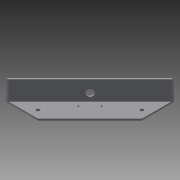
# Autodesk Inventor part: body_inner_L_clamp
Saved by Autodesk Inventor 2015 (Build 190159000, 159)
## iProperties
Created: 2017-09-26
Part Number: body_inner_L_clamp
Material: Generic
Document SubType Name: Modeling
Designer: Anshul
Density: 1 g/cm^3
Appearance: Default
Author: Anshul
Autodesk Inventor part; units mm, degrees
ref_plane "YZ Plane" through (0, 0, 0) normal (1, 0, 0) x (0, 1, 0)
ref_plane "XZ Plane" through (0, 0, 0) normal (0, 1, 0) x (-1, 0, 0)
ref_plane "XY Plane" through (0, 0, 0) normal (0, 0, 1) x (1, 0, 0)
sketch "Sketch1" plane through (0, 0, 0) normal (0, 1, 0) x (-1, 0, 0)
  line L0 (0, 0) -> (0, -650)
  line L1 (0, -650) -> (650, -650)
  line L2 (650, -650) -> (650, 0)
  line L3 (650, 0) -> (0, 0)
  line L4 (0, 0) -> (3, 0)
  line L5 (3, 0) -> (3, -650)
  line L6 (3, -650) -> (0, -650)
  line L7 (0, -650) -> (0, -647)
  line L8 (0, -647) -> (650, -647)
  line L9 (650, -647) -> (650, -650)
  line L10 (650, -650) -> (647, -650)
  line L11 (647, -650) -> (647, 0)
  line L12 (647, 0) -> (650, 0)
  line L13 (650, 0) -> (650, -3)
  line L14 (650, -3) -> (0, -3)
  line L15 (0, -3) -> (0, 0)
  line L16 (0, 0) -> (0, -37)
  line L17 (0, -37) -> (650, -37)
  line L18 (650, -37) -> (650, 0)
  line L19 (650, 0) -> (613, 0)
  line L20 (613, 0) -> (613, -650)
  line L21 (613, -650) -> (650, -650)
  line L22 (650, -650) -> (650, -613)
  line L23 (650, -613) -> (0, -613)
  line L24 (0, -613) -> (0, -650)
  line L25 (0, -650) -> (37, -650)
  line L26 (37, -650) -> (37, 0)
  line L27 (37, 0) -> (0, 0)
  line L28 (0, 0) -> (650, -650)
  line L29 (650, 0) -> (0, -650)
  line L30 (37, -3) -> (3, -37)
  line L31 (20, -20) -> (75.1543, -75.1543)
  line L32 (75.1543, -75.1543) -> (3, -147.3087)
  line L33 (75.1543, -75.1543) -> (147.3087, -3)
  line L34 (75.1543, -75.1543) -> (48.9914, -48.9914)
  line L35 (48.9914, -48.9914) -> (3, -94.9828)
  line L36 (48.9914, -48.9914) -> (94.9828, -3)
  line L37 (75.1543, -75.1543) -> (77.2756, -77.2756)
  line L38 (77.2756, -77.2756) -> (3, -151.5513)
  line L39 (77.2756, -77.2756) -> (151.5513, -3)
  line L40 (75.1543, -75.1543) -> (68.0833, -68.0833)
  line L41 (68.0833, -68.0833) -> (57.8302, -78.3363)
  line L42 (68.0833, -68.0833) -> (78.3363, -57.8302)
  circle A0 centre (78.3363, -57.8302) radius 1.5
  circle A1 centre (57.8302, -78.3363) radius 1.5
  line L43 (3, -147.3087) -> (3, -94.9828)
  line L44 (147.3087, -3) -> (94.9828, -3)
  line L45 (121.1457, -3) -> (3, -121.1457)
  circle A2 centre (62.0729, -62.0729) radius 65
  circle A3 centre (108.0348, -16.1109) radius 3
  circle A4 centre (16.1109, -108.0348) radius 3
  dimension "d0" = 650
  dimension "d1" = 650
  dimension "d2" = 650
  dimension "d3" = 3
  dimension "d4" = 650
  dimension "d5" = 3
  dimension "d6" = 3
  dimension "d7" = 650
  dimension "d8" = 3
  dimension "d9" = 650
  dimension "d10" = 37
  dimension "d11" = 650
  dimension "d12" = 37
  dimension "d13" = 650
  dimension "d14" = 37
  dimension "d15" = 650
  dimension "d16" = 37
  dimension "d17" = 650
  dimension "d18" = 78
  dimension "d19" = 37
  dimension "d20" = 3
  dimension "d21" = 10
  dimension "d22" = 14.5
  dimension "d23" = 14.5
  dimension "d24" = 3
  dimension "d25" = 3
  dimension "d26" = 130
  dimension "d27" = 6
  dimension "d28" = 6
  constraints: 92 end point, 35 point on line, 8 perpendicular, 5 centre point, 5 collinear, 4 midpoint, 2 coincident, 2 point on circle, 1 parallel, 1 vertical
  measures "d0" distance of L0.start L0.end
  measures "d1" distance of L0.end L1.end
  measures "d2" distance of L1.end L2.end
  measures "d3" distance of L0.start L4.end
  measures "d4" distance of L4.end L5.end
  measures "d5" distance of L0.end L7.end
  measures "d6" distance of L1.end L10.end
  measures "d7" distance of L10.end L11.end
  measures "d8" distance of L2.end L13.end
  measures "d9" distance of L13.end L14.end
  measures "d10" distance of L0.start L16.end
  measures "d11" distance of L16.end L17.end
  measures "d12" distance of L2.end L19.end
  measures "d13" distance of L19.end L20.end
  measures "d14" distance of L1.end L22.end
  measures "d15" distance of L22.end L23.end
  measures "d16" distance of L0.end L25.end
  measures "d17" distance of L25.end L26.end
  measures "d18" distance of L31.start L31.end
  measures "d19" distance of L31.end L34.end
  measures "d20" distance of L31.end L37.end
  measures "d21" distance of L31.end L40.end
  measures "d22" distance of L40.end L41.end
  measures "d23" distance of L40.end L42.end
  measures "d24" diameter of A0
  measures "d25" diameter of A1
  measures "d26" diameter of A2
  measures "d27" diameter of A3
  measures "d28" diameter of A4
extrude "Extrusion1" add sketch "Sketch1" along normal blind 3 contours L35 A2 A4 L45 L5 | L35 L26 L45 A4 A2 | L36 A2 A3 L45 L17 | L17 L45 L28 L36 | L35 L28 L45 L26 | L14 L45 A3 A2 L36 | L45 A4 A2 L32 L5 | L45 A3 A2 L33 L17 | L17 L33 L28 L45 | L45 L28 L32 L26 | L26 L32 A2 A4 L45 | L14 L33 A2 A3 L45
extrude "Extrusion2" add sketch "Sketch1" along normal blind 37 contours L5 L32 A2 L38 | L39 A2 L33 L14 | L33 A2 L39 L17 | L17 L39 L28 L33 | L32 L28 L38 L26 | L26 L38 A2 L32
sketch "Sketch2" plane through (-151.5513, 0, -3) normal (-0.7071, 0, -0.7071) x (-0.7071, 0, 0.7071)
  line L0 (-105.0416, 0) -> (-105.0416, 3)
  line L1 (-105.0416, 3) -> (-105.0416, 23)
  line L2 (-3, 37) -> (-207.0833, 37) projected
  line L3 (-105.0416, 23) -> (-105.0416, 16)
  circle A0 centre (-105.0416, 16) radius 6
  dimension "d33" = 3
  dimension "d39" = 20
  dimension "d40" = 7
  dimension "d41" = 12
  constraints: 6 end point, 1 centre point, 1 coincident, 1 perpendicular, 1 point on line, 1 vertical
  measures "d33" distance of L0.start L0.end
  measures "d39" distance of L0.end L1.end
  measures "d40" distance of L1.end L3.end
  measures "d41" diameter of A0
extrude "Extrusion4" cut sketch "Sketch2" against normal blind 10
body "Solid1"
